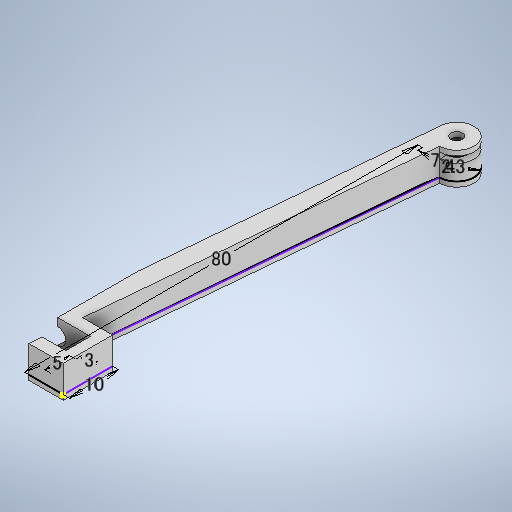
# Autodesk Inventor part: srod1
Saved by Autodesk Inventor 2025 (Build 290162000, 162)
## iProperties
Created: 2024-07-27
Part Number: srod1
Material: 一般
Document SubType Name: Modeling
Designer: Saigusa
Density: 1 g/cm^3
Appearance: 既定
Author: Saigusa
Autodesk Inventor part; units mm, degrees
ref_plane "YZ Plane" through (0, 0, 0) normal (1, 0, 0) x (0, 1, 0)
ref_plane "XZ Plane" through (0, 0, 0) normal (0, 1, 0) x (-1, 0, 0)
ref_plane "XY Plane" through (0, 0, 0) normal (0, 0, 1) x (1, 0, 0)
sketch "スケッチ1" plane through (0, 0, 0) normal (0, 1, 0) x (-1, 0, 0)
  circle A0 centre (0, 0) radius 1.15
  circle A1 centre (0, 0) radius 2
  circle A2 centre (0, 0) radius 3.5
  line L0 (0, 0) -> (0, 3.5)
  line L1 (2, 0) -> (2, -2.8723)
  line L2 (-2, 0) -> (-2, -2.8723)
  line L3 (0, 0) -> (3.5, 0)
  line L4 (3.5, 0) -> (3.5, 3.5)
  line L5 (3.5, 3.5) -> (0, 3.5)
  line L6 (0, 3.5) -> (0, 0)
  line L7 (0, 0) -> (7, 0)
  line L8 (7, 0) -> (7, 80)
  line L9 (7, 80) -> (0, 0)
  line L10 (0, 3.5) -> (7, 80)
  line L11 (3.5, 0) -> (7, 38.25)
  line L12 (7, 80) -> (0, 80)
  line L13 (0, 80) -> (0, 70)
  line L14 (0, 70) -> (7, 70)
  line L15 (3.5, 80) -> (3.5, 70)
  line L16 (2, 77.5) -> (5, 77.5)
  line L17 (5, 77.5) -> (5, 72.5)
  line L18 (5, 72.5) -> (2, 72.5)
  line L19 (2, 72.5) -> (2, 77.5)
  line L20 (2, 77.5) -> (5, 72.5) construction
  line L21 (5, 77.5) -> (2, 72.5) construction
  line L22 (2, 72.5) -> (7, 72.5)
  line L23 (2, 77.5) -> (7, 77.5)
  point P0 (0, 2)
  point P1 (3.5, 75)
  point P2 (6.3438, 72.5)
  point P3 (6.125, 70)
  point P4 (6.085, 70)
  point P5 (0.3063, 3.5)
  point P6 (0.3051, 3.4867)
  point P7 (6.3137, 72.5)
  point P8 (6.7712, 77.5)
  dimension "d0" = 2.3
  dimension "d1" = 4
  dimension "d2" = 7
  dimension "d11" = 7
  dimension "d12" = 80
  dimension "d13" = 10
  dimension "d14" = 3
  dimension "d15" = 5
  constraints: 48 end point, 8 parallel, 6 point on line, 5 midpoint, 5 point on circle, 4 horizontal, 4 perpendicular, 3 centre point, 3 coincident, 1 tangent, 1 vertical
  measures "d0" diameter of A0
  measures "d1" diameter of A1
  measures "d2" diameter of A2
  measures "d11" distance of L0.start L7.end
  measures "d12" distance of L7.end L8.end
  measures "d13" distance of L12.end L13.end
  measures "d14" distance of L17.end L18.end
  measures "d15" distance of L16.end L17.end
extrude "押し出し1" add sketch "スケッチ1" along normal blind 3.2 contours A1 L2 A2 L0
extrude "押し出し2" add sketch "スケッチ1" along normal blind 4.5 contours L3 A2 L1 | A1 L9 A2 L3 | A1 L0 A2 L9
extrude "押し出し3" add sketch "スケッチ1" against normal blind 1 contours L3 A1 L0 A0 | A0 L9 A1 L3 | A0 L0 A1 L9 | L1 A2 L2 A1 | L3 A2 L1 | A1 L9 A2 L3 | A1 L0 A2 L9 | A1 L2 A2 L0
sketch "スケッチ3" plane through (0, 4.5, 0) normal (0, 1, 0) x (1, 0, 0)
  circle A0 centre (0, 0) radius 1.15
  circle A1 centre (0, 0) radius 2
  circle A2 centre (0, 0) radius 3.5
  dimension "d17" = 2.3
  dimension "d18" = 4
  dimension "d19" = 7
  constraints: 3 centre point, 3 coincident
  measures "d17" diameter of A0
  measures "d18" diameter of A1
  measures "d19" diameter of A2
extrude "押し出し5" add sketch "スケッチ3" along normal blind 1 contours A1 | A2
extrude "押し出し6" add sketch "スケッチ1" along normal blind 5.5 contours A2 L9 L5 L4 | L4 L5 L9 L14 L8 L11 | A2 L5 L9 | L10 L14 L9 L5 | L14 L15 L18 L22 L10 | L10 L22 L9 L14 | L14 L9 L22 L8 | L14 L13 L12 L15 L16 L19 L18 | L23 L16 L15 L12 L10
extrude "押し出し7" add sketch "スケッチ1" against normal blind 1 contours A2 L9 L5 L4 | L4 L5 L9 L14 L8 L11 | L10 L14 L9 L5 | L14 L15 L18 L22 L10 | L10 L22 L9 L14 | L14 L9 L22 L8 | L14 L13 L12 L15 L16 L19 L18 | L23 L16 L15 L12 L10
sketch "スケッチ5" plane through (-7, 5.5, 72.5) normal (0, 0, 1) x (1, 0, 0)
  line L0 (0.2288, 0) -> (0, 0) projected
  line L1 (0, 0) -> (0, -3.25)
  line L2 (5, -6.5) -> (0, -6.5) projected
  line L3 (0, -3.25) -> (-1.65, -3.25)
  circle A0 centre (-1.65, -3.25) radius 1.65
  line L4 (-1.65, -3.25) -> (-1.65, 0)
  line L5 (-1.65, 0) -> (-1.65, -6.5)
  line L6 (-1.65, -6.5) -> (0, -6.5)
  line L7 (-1.65, 0) -> (0, 0)
  line L8 (0, -6.5) -> (0, 0) projected
  line L9 (0, -3.25) -> (0, -6.5)
  point P0 (7, -5.5)
  point P1 (-1.65, -4.9)
  point P2 (-1.65, -1.6)
  dimension "d28" = 3.25
  dimension "d29" = 1.65
  constraints: 14 end point, 2 collinear, 2 perpendicular, 1 coincident, 1 horizontal, 1 point on line, 1 vertical, 3 other
  measures "d28" distance of L0.end L1.end
  measures "d29" distance of L1.end L3.end
extrude "押し出し8" add sketch "スケッチ5" against normal up to surface contours L1 A0 L4 L7 | L8 L6 L5 A0 surface through (-3.5, 0, 0) normal (-0.9958, 0, -0.0911)
sketch "スケッチ6" plane through (-7, 5.5, 80) normal (0, 0, 1) x (1, 0, 0)
  point P0 (7, -5.5)
